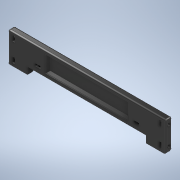
# Autodesk Inventor part: Lateral
Saved by Autodesk Inventor 2020 (Build 240168000, 168)
## iProperties
Created: 2021-06-24
Part Number: Lateral
Material: Genérico
Document SubType Name: Modeling
Designer: JCarlos
Density: 1 g/cm^3
Appearance: Brilhosa - Preta
Author: JCarlos
Autodesk Inventor part; units mm, degrees
ref_plane "YZ Plane" through (0, 0, 0) normal (1, 0, 0) x (0, 1, 0)
ref_plane "XZ Plane" through (0, 0, 0) normal (0, 1, 0) x (-1, 0, 0)
ref_plane "XY Plane" through (0, 0, 0) normal (0, 0, 1) x (1, 0, 0)
sketch "Esboço1" plane through (0, 0, 0) normal (0, 0, 1) x (1, 0, 0)
  line L0 (-80, 15) -> (80, 15)
  line L1 (80, 15) -> (80, -15)
  line L2 (80, -15) -> (-80, -15)
  line L3 (-80, -15) -> (-80, 15)
  point P0 (0, 0)
  point P1 (-80, 0)
  point P2 (0, 15)
  dimension "d0" = 160
  dimension "d1" = 30
  constraints: 8 end point, 2 midpoint, 2 parallel, 1 horizontal, 1 horizontal alignment, 1 perpendicular, 1 vertical alignment
  measures "d0" distance of L0.start L0.end
  measures "d1" distance of L2.end L0.start
extrude "Extrusão1" add sketch "Esboço1" along normal blind 6.5
sketch "Esboço2" plane through (80, -15, 0) normal (1, 0, 0) x (0, 0, -1)
  circle A0 centre (-3.25, 24.5) radius 1.75
  circle A1 centre (-3.25, 5.5) radius 1.75
  line L0 (-6.5, 0) -> (-6.5, 30) projected
  point P0 (0, 15)
  dimension "d4" = 3.5
  dimension "d5" = 19
  dimension "d6" = 9.5
  dimension "d7" = 3.25
  constraints: 2 centre point, 1 equal radius, 1 vertical alignment
  measures "d4" diameter of A0
  measures "d5" distance of A1.centre A0.centre
  measures "d6" vertical distance of point (0, 15) A0.centre
  measures "d7" distance from line of L0 A0.centre
extrude "Extrusão2" cut sketch "Esboço2" against normal blind 10
sketch "Esboço3" plane through (0, 0, 6.5) normal (0, 0, 1) x (1, 0, 0)
  line L0 (73, 6.65) -> (75.7, 6.65)
  line L1 (75.7, 6.65) -> (75.7, 12.35)
  line L2 (75.7, 12.35) -> (73, 12.35)
  line L3 (73, 12.35) -> (73, 6.65)
  line L4 (73, -6.65) -> (75.7, -6.65)
  line L5 (75.7, -6.65) -> (75.7, -12.35)
  line L6 (75.7, -12.35) -> (73, -12.35)
  line L7 (73, -12.35) -> (73, -6.65)
  line L8 (80, 11.25) -> (80, 7.75) projected
  line L9 (80, -7.75) -> (80, -11.25) projected
  line L10 (80, -15) -> (80, 15) projected
  point P0 (0, 0)
  point P1 (75.7, 9.5)
  point P2 (80, 9.5)
  point P3 (75.7, -9.5)
  point P4 (80, -9.5)
  dimension "d10" = 2.7
  dimension "d11" = 5.7
  dimension "d40" = 7
  constraints: 16 end point, 4 midpoint, 4 parallel, 2 horizontal, 2 horizontal alignment, 2 perpendicular, 2 point on line, 1 collinear
  measures "d10" distance of L0.start L0.end
  measures "d11" distance of L2.end L0.start
  measures "d40" distance between parallel lines of L3 L10
extrude "Extrusão3" cut sketch "Esboço3" against normal through all
mirror "Espelhamento1" about plane through (0, 0, 0) normal (1, 0, 0) of "Extrusão2", "Extrusão3"
sketch "Esboço5" plane through (0, 0, 6.5) normal (0, 0, 1) x (1, 0, 0)
  line L0 (-80, -15) -> (80, -15) projected
  line L1 (-60.25, -15) -> (60.25, -15)
  line L2 (60.25, -15) -> (60.25, -8)
  line L3 (60.25, -8) -> (-60.25, -8)
  line L4 (-60.25, -8) -> (-60.25, -15)
  point P0 (0, 0)
  point P1 (0, -8)
  dimension "d15" = 7
  dimension "d16" = 120.5
  constraints: 8 end point, 2 parallel, 1 horizontal, 1 midpoint, 1 perpendicular, 1 point on line, 1 vertical alignment
  measures "d15" distance of L3.end L1.start
  measures "d16" distance of L2.end L3.end
extrude "Extrusão4" cut sketch "Esboço5" against normal through all
sketch "Esboço6" plane through (-60.25, -8, 6.5) normal (0, -1, 0) x (1, 0, 0)
  circle A0 centre (110.25, -3.25) radius 1.75
  line L0 (140.25, -6.5) -> (140.25, 0) projected
  line L1 (120.5, 0) -> (120.5, -6.5) projected
  point P0 (60.25, -6.5)
  point P1 (140.25, -3.25)
  dimension "d19" = 3.5
  dimension "d38" = 50
  constraints: 1 centre point, 1 horizontal alignment, 1 midpoint
  measures "d19" diameter of A0
  measures "d38" horizontal distance of point (60.25, -6.5) A0.centre
extrude "Extrusão5" cut sketch "Esboço6" against normal blind 10
sketch "Esboço7" plane through (0, 0, 6.5) normal (0, 0, 1) x (1, 0, 0)
  line L0 (47.15, -1) -> (52.85, -1)
  line L1 (52.85, -1) -> (52.85, -3.7)
  line L2 (52.85, -3.7) -> (47.15, -3.7)
  line L3 (47.15, -3.7) -> (47.15, -1)
  line L4 (51.75, -8) -> (48.25, -8) projected
  point P0 (0, 0)
  point P1 (50, -3.7)
  point P2 (50, -8)
  dimension "d23" = 5.7
  dimension "d24" = 2.7
  dimension "d41" = 7
  constraints: 8 end point, 2 midpoint, 2 parallel, 1 horizontal, 1 perpendicular, 1 vertical alignment
  measures "d23" distance of L0.start L0.end
  measures "d24" distance of L0.end L1.end
  measures "d41" distance between parallel lines of L4 L0
extrude "Extrusão6" cut sketch "Esboço7" against normal through all
mirror "Espelhamento2" about plane through (0, 0, 0) normal (1, 0, 0) of "Extrusão5", "Extrusão6"
sketch "Esboço8" plane through (0, 0, 6.5) normal (0, 0, 1) x (1, 0, 0)
  line L0 (-42.15, 12) -> (42.15, 12)
  line L1 (42.15, 12) -> (42.15, -5)
  line L2 (42.15, -5) -> (-42.15, -5)
  line L3 (-42.15, -5) -> (-42.15, 12)
  line L4 (80, 15) -> (-80, 15) projected
  line L5 (-60.25, -8) -> (60.25, -8) projected
  line L6 (-47.15, -1) -> (-47.15, -3.7) projected
  line L7 (47.15, -3.7) -> (47.15, -1) projected
  point P0 (0, 0)
  dimension "d28" = 3
  dimension "d29" = 3
  dimension "d30" = 5
  dimension "d31" = 5
  constraints: 8 end point, 2 parallel, 1 horizontal, 1 perpendicular
  measures "d28" distance between parallel lines of L4 L0
  measures "d29" distance between parallel lines of L5 L2
  measures "d30" distance between parallel lines of L6 L3
  measures "d31" distance between parallel lines of L7 L1
extrude "Extrusão7" cut sketch "Esboço8" against normal blind 3
fillet "Arredondamento1" radius 1.5 10 edges at (-80, 15, 3.25) (80, 15, 3.25) (0, 15, 6.5) (0, 15, 0) (-80, 0, 6.5) (-80, 0, 0) (80, 0, 6.5) (80, 0, 0) (80, -15, 3.25) (-80, -15, 3.25)
chamfer "Chanfro1" distance 2 angle 45 4 edges at (0, 12, 3.5) (-42.15, 3.5, 3.5) (42.15, 3.5, 3.5) (0, -5, 3.5)
fillet "Arredondamento2" radius 2 4 edges at (-79.5607, -14.5607, 0.4393) (-69.3751, -15, 0) (79.5607, -14.5607, 0.4393) (69.375, -15, 0)
equation "\"d6\" = 0.5 * d5"
equation "\"d7\" = 0.5 * d2"
equation "\"d29\" = d28"
equation "\"d2\" = 6.5"
